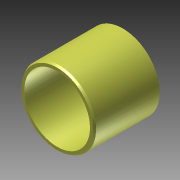
# Autodesk Inventor part: JSI-1618-16
Saved by Autodesk Inventor 2011 (Build 150239000, 239)
## iProperties
Category: Plastic Bearings
Created: 2007-11-11
Part Number: JSI-1618-16
Material: iglide J
Catalog Web Link: http://www.igus.com/igubal/igl3.asp?x=JSI-1618-16
Description: iglide J Sleeve Bearing
Vendor: igus
Document SubType Name: Modeling
Mass: 5.8346 g
Surface Area: 52.0262 cm^2
Volume: 3.91584 cm^3
Density: 1.49 g/cm^3
Project: FIRST
Title: iglide J Sleeve Bearing
Author: Autodesk, Inc.
Autodesk Inventor part; units mm, degrees
ref_plane "YZ Plane" through (0, 0, 0) normal (1, 0, 0) x (0, 1, 0)
ref_plane "XZ Plane" through (0, 0, 0) normal (0, 1, 0) x (-1, 0, 0)
ref_plane "XY Plane" through (0, 0, 0) normal (0, 0, 1) x (1, 0, 0)
sketch "Sketch1" plane through (0, 0, 0) normal (0, 0, 1) x (1, 0, 0)
  circle A0 centre (0, 0) radius 14.2875
  dimension "d0" = 28.575
  constraints: 1 centre point, 1 coincident
  measures "d0" diameter of A0
extrude "Body" add sketch "Sketch1" along normal blind 25.4
hole "Hole" at (0, 0, 25.4) direction (0, 0, -1) diameter 25.4 end through all
chamfer "Chamfer - Outside" distance 0.7874 angle 30 1 edges at (-14.2875, 0, 25.4) measured on face at (14.2412, -1.1497, 16.9333)
chamfer "Chamfer - Inside" distance 0.7874 angle 30 1 edges at (0, 12.7, 0) measured on face at (1.0219, -12.6588, 16.9333)
body "Solid1"
